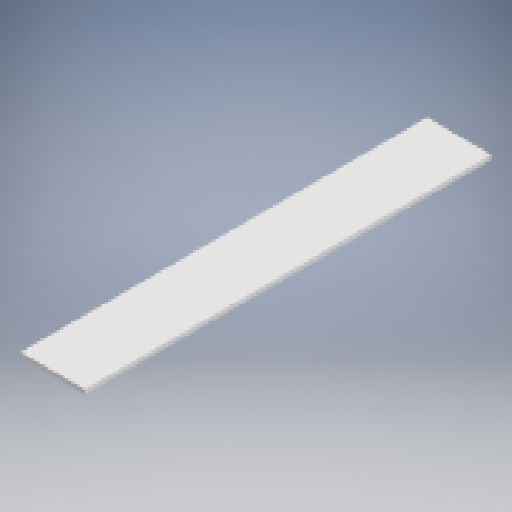
# Autodesk Inventor part: SIDE SH2
Saved by Autodesk Inventor 2025.2 (Build 292293000, 293)
## iProperties
Created: 2025-01-29
Part Number: SIDE SH2
Material: Wood (Birch)
Document SubType Name: Modeling
Designer: Anna
Density: 0.55 g/cm^3
Appearance: Birch - Natural Polished
Mass: 5167.76 g
Surface Area: 10643.5 cm^2
Volume: 9395.93 cm^3
Author: Anna
Autodesk Inventor part; units mm, degrees
ref_plane "YZ Plane" through (0, 0, 0) normal (1, 0, 0) x (0, 1, 0)
ref_plane "XZ Plane" through (0, 0, 0) normal (0, 1, 0) x (-1, 0, 0)
ref_plane "XY Plane" through (0, 0, 0) normal (0, 0, 1) x (1, 0, 0)
sketch "Sketch1" plane through (0, 0, 0) normal (1, 0, 0) x (0, 1, 0)
  line L0 (0, 431.8) -> (0, -431.8)
  line L1 (0, 431.8) -> (19.05, 431.8)
  line L2 (19.05, 431.8) -> (19.05, -431.8)
  line L3 (19.05, -431.8) -> (0, -431.8)
  point P0 (0, 0)
  dimension "d0" = 863.6
  dimension "d1" = 19.05
  constraints: 8 end point, 2 perpendicular, 1 horizontal, 1 midpoint, 1 vertical
  measures "d0" distance of L0.start L0.end
  measures "d1" distance of L0.start L1.end
extrude "Extrusion1" add sketch "Sketch1" along normal blind 279.4
body "Solid1"
